Autodesk Fusion 360 part; units mm, degrees
(part 2 of 2)
sketch "Left heatsink lock profile" plane through (-24.1, 0, 0) normal (1, 0, 0) x (0, 1, 0) in component "Heatsink locks"
  line L0 (-5, 8) -> (29.1, 8)
  line L1 (29.1, 8) -> (29.1, 14)
  line L2 (29.1, 14) -> (-5, 14)
  line L3 (-5, 14) -> (-5, 8)
  line L4 (8, 8) -> (8, 18.5306) construction
  line L5 (31.1324, 10) -> (-6.2812, 10) construction
  circle A0 centre (8, 11.5) radius 1.5
  line L6 (9.5, 11.5) -> (9.5, 8)
  line L7 (6.5, 11.5) -> (6.5, 8)
  line L8 (-5, 10) -> (4.6569, 14)
  line L9 (-5, 10) -> (6.7297, 10) construction
  line L10 (29.1, 10) -> (19.4431, 14)
  line L11 (29.1, 10) -> (40.9438, 10) construction
  point P0 (29.1, 8)
  dimension "d129" = 2
  dimension "d130" = 3
  dimension "d131" = 3.5
  dimension "d132" = 22.5
  dimension "d133" = 157.5
  constraint coincident L0 L4.start
  constraint perpendicular L0 L4
  constraint perpendicular L3 L5
  constraint coincident L4 A0.centre
  constraint coincident L0 L6.end
  constraint perpendicular L0 L6
  constraint coincident L0 L7.end
  constraint perpendicular L0 L7
  constraint tangent A0 L7
  constraint tangent A0 L6
  constraint coincident A0 L7.start
  constraint coincident A0 L6.start
  constraint horizontal L9
  constraint coincident L3 L8.start
  constraint coincident L5 L8.start
  constraint coincident L2 L8.end
  constraint horizontal L11
  constraint coincident L5 L10.start
  constraint coincident L1 L10.start
  constraint coincident L2 L10.end
  measures "d129" vertical distance of L5.start P0
  measures "d130" diameter of A0
  measures "d131" distance of L4.start A0.centre
  measures "d132" angle of L8 L9
  measures "d133" angle of L10 L11
sketch "Screw head countersinks" plane through (0, 0, 14) normal (0, 0, 1) x (-1, 0, 0) in component "Heatsink locks"
  circle A0 centre (34.0203, 0.0351) radius 1.5
  circle A1 centre (26.7388, -23.0505) radius 1.5
  line L0 (38.2285, 0.0793) -> (36.5619, 5)
  line L1 (36.5619, 5) -> (24.1, 5)
  line L2 (24.1, 5) -> (24.1, -29.1)
  line L3 (24.1, -29.1) -> (29.025, -29.1)
  line L4 (29.025, -29.1) -> (38.2285, 0.0793)
  circle A2 centre (34.0203, 0.0351) radius 2.75
  circle A3 centre (26.7388, -23.0505) radius 2.75
  circle A4 centre (-28.498, 0) radius 2.75
  circle A5 centre (-26.9591, 22.8364) radius 2.75
extrude "Extrude2''" cut sketch "Screw head countersinks" against normal blind 4 contours L2 A3 | A2 | A4 | A5 picked at (24.4796, -23.0505) bodies 7 8 in component "Heatsink locks"
extrude "Extrude3'" cut sketch "Left heatsink lock profile" against normal blind 17 contours L0 A0 L6 L7 | L2 L3 L8 | A0 | L1 L2 L10 bodies 7 in component "Heatsink locks"
sketch "Right heatsink lock profile" plane through (24.1, 0, 0) normal (-1, 0, 0) x (0, -1, 0) in component "Heatsink locks"
  line L0 (-5, 8) -> (29.1, 8)
  line L1 (29.1, 8) -> (29.1, 14)
  line L2 (29.1, 14) -> (-5, 14)
  line L3 (-5, 14) -> (-5, 8)
  line L4 (8, 8) -> (8, 20) construction
  line L5 (31.5717, 10) -> (-7.4044, 10) construction
  line L6 (-5, 10) -> (4.6569, 14)
  line L7 (-5, 10) -> (7.1624, 10) construction
  line L8 (29.1, 10) -> (19.4431, 14)
  line L9 (29.1, 10) -> (41.2336, 10) construction
  circle A0 centre (8, 11.5) radius 1.5
  line L10 (9.5, 11.5) -> (9.5, 8)
  line L11 (6.5, 11.5) -> (6.5, 8)
  point P0 (29.1, 8)
  point P1 (8, 8)
  dimension "d138" = 2
  dimension "d139" = 22.5
  dimension "d140" = 157.5
  dimension "d141" = 3
  dimension "d142" = 3.5
  constraint coincident L0 P1
  constraint perpendicular L2 L4
  constraint horizontal L5
  constraint horizontal L7
  constraint coincident L3 L6.start
  constraint coincident L5 L6.start
  constraint coincident L2 L6.end
  constraint horizontal L9
  constraint coincident L5 L8.start
  constraint coincident L1 L8.start
  constraint coincident L2 L8.end
  constraint coincident L4 A0.centre
  constraint coincident L0 L10.end
  constraint perpendicular L0 L10
  constraint coincident L0 L11.end
  constraint perpendicular L0 L11
  constraint tangent A0 L11
  constraint tangent A0 L10
  constraint coincident A0 L11.start
  constraint coincident A0 L10.start
  measures "d138" vertical distance of L5.start P0
  measures "d139" angle of L6 L7
  measures "d140" angle of L8 L9
  measures "d141" diameter of A0
  measures "d142" distance of A0.centre P1
extrude "Extrude4'" cut sketch "Right heatsink lock profile" against normal blind 16 contours L0 A0 L10 L11 | L2 L3 L6 | A0 | L1 L2 L8 bodies 8 in component "Heatsink locks"
component "Bottom frame" placed x (1, 0, 0) y (0, 1, 0) z (0, 0, 1) at (0, 0, 0)
component "Top frame" placed x (1, 0, 0) y (0, 1, 0) z (0, 0, 1) at (0, 0, 0)
component "Heatsink locks" placed x (1, 0, 0) y (0, 1, 0) z (0, 0, 1) at (0, 0, 0)
equation "d27 = d24"
equation "d33 = d24"
equation "d34 = d24"
equation "d35 = d24"
equation "d41 = d24"
equation "d42 = d41"
equation "d43 = d41"
equation "d44 = d42"
equation "d45 = d44"
equation "d46 = d45"
equation "d58 = d57"
equation "d59 = d57"
equation "d60 = d57"
equation "d61 = d57"
equation "d63 = d62"
equation "d64 = d62 / 2"
equation "d65 = d64"
equation "d67 = d66"
equation "d68 = d66"
equation "d69 = d66"
equation "d70 = d66"
equation "d72 = d71"
equation "d73 = d71"
equation "d74 = d71"
equation "d75 = d71"
equation "d81 = d80"
equation "d82 = d80"
equation "d83 = d80"
equation "d84 = d80"
equation "d92 = d91"
equation "d94 = d91 / 2"
equation "d95 = d94"
equation "d99 = d96"
equation "d100 = d97"
equation "d101 = d98"
equation "d102 = d96"
equation "d103 = d97"
equation "d104 = d98"
equation "d105 = d96"
equation "d106 = d97"
equation "d107 = d98"
equation "d108 = d96"
equation "d109 = d97"
equation "d110 = d98"
equation "d111 = ( 2.54 * 2 ) * 1 mm"
equation "d112 = ( 2.54 / 2 ) * 1 mm"
equation "d113 = ( 2.54 / 2 ) * 1 mm"
equation "d117 = d116"
equation "d131 = 5 mm - 1.5 mm"
equation "d133 = 180 deg - 22.5 deg"
equation "d140 = 180 deg - 22.5 deg"
equation "d142 = 5 mm - 1.5 mm"
named bodies: "Bottom frame", "Top frame", "Left heatsink lock", "Right heatsink lock"
